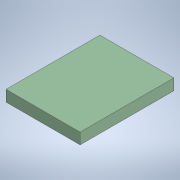
# Autodesk Inventor part: MotorDriverShield
Saved by Autodesk Inventor 2022.2 (Build 262287010, 287A)
## iProperties
Created: 2022-03-26
Part Number: MotorDriverShield
Material: Generic
Document SubType Name: Modeling
Designer: Santiago Larraín
Density: 1 g/cm^3
Appearance: Default
Author: Santiago Larraín
Autodesk Inventor part; units mm, degrees
ref_plane "YZ Plane" through (0, 0, 0) normal (1, 0, 0) x (0, 1, 0)
ref_plane "XZ Plane" through (0, 0, 0) normal (0, 1, 0) x (-1, 0, 0)
ref_plane "XY Plane" through (0, 0, 0) normal (0, 0, 1) x (1, 0, 0)
sketch "Sketch1" plane through (0, 0, 0) normal (0, 1, 0) x (-1, 0, 0)
  line L0 (0, 0) -> (0, -65)
  line L1 (0, -65) -> (51.3, -65)
  line L2 (51.3, -65) -> (51.3, 0)
  line L3 (51.3, 0) -> (0, 0)
  dimension "d0" = 65
  dimension "d1" = 51.3
  constraints: 8 end point, 2 parallel, 1 perpendicular, 1 vertical
  measures "d0" distance of L0.start L0.end
  measures "d1" distance of L1.end L0.end
extrude "Extrusion1" add sketch "Sketch1" along normal blind 7.675
body "Solid1"
